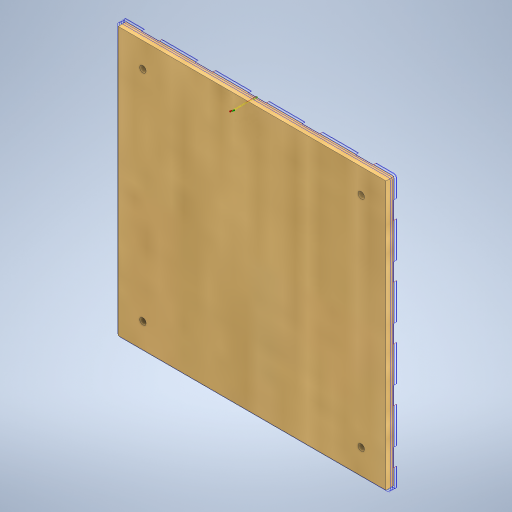
# Autodesk Inventor part: Tapa_abajo
Saved by Autodesk Inventor 2023 (Build 270158000, 158)
## iProperties
Created: 2022-12-03
Part Number: Tapa_abajo
Material: Genérico
Document SubType Name: Modeling
Designer: sergi
Density: 1 g/cm^3
Appearance: Valor por defecto
Author: sergi
Autodesk Inventor part; units mm, degrees
ref_plane "YZ Plane" through (0, 0, 0) normal (1, 0, 0) x (0, 1, 0)
ref_plane "XZ Plane" through (0, 0, 0) normal (0, 1, 0) x (-1, 0, 0)
ref_plane "XY Plane" through (0, 0, 0) normal (0, 0, 1) x (1, 0, 0)
sketch "Boceto1" plane through (0, 0, 0) normal (0, 0, 1) x (1, 0, 0)
  line L0 (-1.5, -51.5) -> (-1.5, 51.5)
  line L1 (98.5, -51.5) -> (18.2, -51.5)
  line L2 (101.5, 51.5) -> (101.5, -51.5)
  line L3 (101.5, -51.5) -> (-1.5, -51.5)
  line L4 (-1.5, -51.5) -> (-1.5, 51.5)
  line L5 (-1.5, 51.5) -> (101.5, 51.5)
  line L6 (101.5, 51.5) -> (101.5, -51.5)
  circle A0 centre (8, -42) radius 1.25
  circle A1 centre (8, 42) radius 1.25
  circle A2 centre (92, 42) radius 1.25
  circle A3 centre (92, -42) radius 1.25
  point P0 (0, 0)
extrude "Extrusión1" add sketch "Boceto1" along normal blind 3
